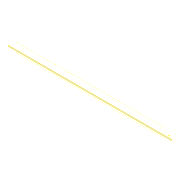
# Autodesk Inventor part: Bearing mount for xrail
Saved by Autodesk Inventor 2020 (Build 240168000, 168)
## iProperties
Created: 2019-12-20
Part Number: Bearing mount for xrail
Material: Generic
Document SubType Name: Modeling
Designer: ball
Density: 1 g/cm^3
Appearance: Default
Author: ball
Autodesk Inventor part; units mm, degrees
ref_plane "YZ Plane" through (0, 0, 0) normal (1, 0, 0) x (0, 1, 0)
ref_plane "XZ Plane" through (0, 0, 0) normal (0, 1, 0) x (-1, 0, 0)
ref_plane "XY Plane" through (0, 0, 0) normal (0, 0, 1) x (1, 0, 0)
ref_plane "Work Plane1" through (0, 0, 0) normal (0, 0, 1) x (1, 0, 0)
sketch "Sketch1" plane through (0, 0, 0) normal (0, 0, 1) x (1, 0, 0)
  line L0 (-9.7566, -4.627) -> (-9.7566, 4.627) construction
  line L1 (-9.7566, -9.525) -> (-314.5566, -9.525) construction
  line L2 (-9.7566, 9.525) -> (-314.5566, 9.525) construction
  line L3 (-42.7766, 3) -> (-42.7766, -3) construction
  line L4 (-9.7566, 9.525) -> (-42.7766, 9.525)
  line L5 (-42.7766, 9.525) -> (-42.7766, -9.525)
  line L6 (-9.7566, -9.525) -> (-9.7566, 9.525)
  line L7 (-9.7566, -9.525) -> (-9.7566, -28.575)
  line L8 (-9.7566, -28.575) -> (-42.7766, -28.575)
  line L9 (-42.7766, -28.575) -> (-42.7766, -9.525)
  arc A0 (-38.0982, 0.6213) -> (-38.1469, -0.737) centre (-39.737, 0) ccw construction
  arc A1 (-11.1575, 0.6213) -> (-11.2061, -0.737) centre (-12.7962, 0) ccw construction
  circle A2 centre (-12.7962, 0) radius 1.9304
  circle A3 centre (-39.737, 0) radius 1.9304
  point P0 (0, 0)
  dimension "d1" = 19.05
  dimension "d2" = 3.8608
  dimension "d3" = 3.8608
  constraints: 12 end point, 2 centre point, 2 coincident, 2 parallel, 1 horizontal, 1 perpendicular, 1 point on line
  measures "d1" distance of L7.start L7.end
  measures "d2" diameter of A2
  measures "d3" diameter of A3
extrude "Extrusion1" add sketch "Sketch1" along normal blind 5.08
body "Solid1"
